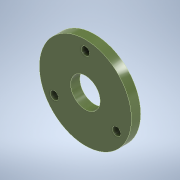
# Autodesk Inventor part: Retentor
Saved by Autodesk Inventor 2021 (Build 250183000, 183)
## iProperties
Created: 2021-04-08
Part Number: Retentor
Material: Genérico
Document SubType Name: Modeling
Designer: rubia
Density: 1 g/cm^3
Appearance: Oliva escuro
Author: rubia
Autodesk Inventor part; units mm, degrees
ref_plane "YZ Plane" through (0, 0, 0) normal (1, 0, 0) x (0, 1, 0)
ref_plane "XZ Plane" through (0, 0, 0) normal (0, 1, 0) x (-1, 0, 0)
ref_plane "XY Plane" through (0, 0, 0) normal (0, 0, 1) x (1, 0, 0)
sketch "Esboço1" plane through (0, 0, 0) normal (0, 0, 1) x (1, 0, 0)
  circle A0 centre (0, 0) radius 25
  circle A1 centre (0, 0) radius 8
  dimension "d0" = 50
  dimension "d1" = 16
  constraints: 2 centre point, 2 coincident
  measures "d0" diameter of A0
  measures "d1" diameter of A1
extrude "Extrusão1" add sketch "Esboço1" along normal blind 5
sketch "Esboço2" plane through (0, 0, 5) normal (0, 0, 1) x (1, 0, 0)
  circle A0 centre (0, 0) radius 14 construction
  circle A1 centre (0, 0) radius 25 construction
  line L0 (0, 25) -> (0, 14) construction
  circle A2 centre (0, 19.5) radius 2.25
  dimension "d4" = 28
  dimension "d5" = 4.5
  constraints: 2 end point, 2 vertical alignment, 1 centre point, 1 coincident, 1 midpoint, 1 vertical, 3 other
  measures "d5" diameter of A2
extrude "Extrusão2" cut sketch "Esboço2" against normal through all
pattern_circular "Padrão circular1" count 3 over 360 about axis through (0, 0, 0) along (0, 0, 1) of "Extrusão2"
